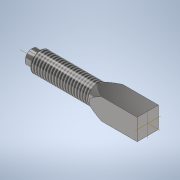
# Autodesk Inventor part: tool clamping screw
Saved by Autodesk Inventor 2021.1 (Build 251245000, 245)
## iProperties
Created: 2021-02-18
Part Number: tool clamping screw
Material: Generic
Document SubType Name: Modeling
Designer: Vamshi
Density: 1 g/cm^3
Appearance: Steel - Polished
Author: Vamshi
Autodesk Inventor part; units mm, degrees
ref_plane "YZ Plane" through (0, 0, 0) normal (1, 0, 0) x (0, 1, 0)
ref_plane "XZ Plane" through (0, 0, 0) normal (0, 1, 0) x (-1, 0, 0)
ref_plane "XY Plane" through (0, 0, 0) normal (0, 0, 1) x (1, 0, 0)
sketch "Sketch1" plane through (0, 0, 0) normal (0, 0, 1) x (1, 0, 0)
  line L0 (0, 0) -> (-81, 0)
  line L1 (-81, 0) -> (-81, 5)
  line L2 (-81, 5) -> (-75, 5)
  line L3 (-75, 5) -> (-75, 7)
  line L4 (-75, 7) -> (-35, 7)
  line L5 (-35, 7) -> (-25, 10.5)
  line L6 (-25, 10.5) -> (0, 10.5)
  line L7 (0, 10.5) -> (0, 0)
  line L8 (-97.2, 0) -> (16.2, 0) projected
  dimension "d7" = 5
  dimension "d8" = 6
  dimension "d9" = 7
  dimension "d10" = 25
  dimension "d11" = 50
  dimension "d12" = 10
  dimension "d13" = 10.5
  constraints: 16 end point, 5 perpendicular, 1 horizontal, 1 parallel
  measures "d7" distance of L0.end L1.end
  measures "d8" distance of L1.end L2.end
  measures "d9" distance between parallel lines of L0 L4
  measures "d10" distance of L5.end L6.end
  measures "d11" horizontal distance of L5.end L3.end
  measures "d12" horizontal distance of L4.end L5.end
  measures "d13" distance of L6.end L0.start
revolve "Revolution1" add sketch "Sketch1" angle 360 about axis through (-10, 0, 0) along (1, 0, 0)
thread "Thread1" size "M14x2" class "6g" standard "ANSI Metric M Profile" full length
sketch "Sketch2" plane through (0, 0, 0) normal (1, 0, 0) x (0, 0, -1)
  circle A0 centre (0, 0) radius 10.5 projected
  line L0 (-7.4246, -7.4246) -> (7.4246, -7.4246)
  line L1 (7.4246, -7.4246) -> (7.4246, 7.4246)
  line L2 (7.4246, 7.4246) -> (-7.4246, 7.4246)
  line L3 (-7.4246, 7.4246) -> (-7.4246, -7.4246)
  line L4 (-7.4246, -7.4246) -> (7.4246, 7.4246) construction
  line L5 (7.4246, -7.4246) -> (-7.4246, 7.4246) construction
  circle A1 centre (0, 0) radius 20.6149
  constraints: 12 end point, 2 midpoint, 2 parallel, 2 perpendicular, 1 centre point, 1 coincident, 1 horizontal, 1 point on circle
extrude "Extrusion1" cut sketch "Sketch2" against normal up to next contours A0 L1 | L2 A0 | A0 L0 | L3 A0 | A1
body "Solid1"
